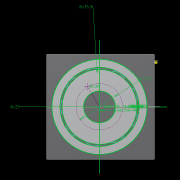
# Autodesk Inventor part: OuterBearingTest_TBS
Saved by Autodesk Inventor 2022.2 (Build 262287010, 287A)
## iProperties
Created: 2022-05-21
Part Number: OuterBearingTest_TBS
Material: Generic
Document SubType Name: Modeling
Designer: Árni Þór Þorgeirsson
Density: 1 g/cm^3
Appearance: Default
Author: Árni Þór Þorgeirsson
Autodesk Inventor part; units mm, degrees
ref_plane "YZ Plane" through (0, 0, 0) normal (1, 0, 0) x (0, 1, 0)
ref_plane "XZ Plane" through (0, 0, 0) normal (0, 1, 0) x (-1, 0, 0)
sketch "Sketch7" plane through (0, 0, 0) normal (0, 1, 0) x (-1, 0, 0)
  line L0 (0, 0) -> (0, 63.4182)
  line L1 (0, 0) -> (-60.766, 0) construction
  line L2 (0, 63.4182) -> (-60.766, 0) construction
  line L3 (0, 63.4182) -> (-66.3755, 0) construction
  line L4 (0, 63.4182) -> (-60.5189, -5.5956) construction
  line L5 (0, 0) -> (0, -63.4182)
  line L6 (0, -63.4182) -> (-60.766, 0) construction
  line L7 (0, -63.4182) -> (-66.3755, 0) construction
  line L8 (0, -63.4182) -> (-60.5189, 5.5956) construction
  line L9 (-60.5189, 5.5956) -> (-66.3755, 0) construction
  line L10 (-55.6121, 0) -> (-64.3632, -8.3612) construction
  line L11 (-55.6121, 0) -> (-39.6464, -15.2543) construction
  line L12 (0, -88.9988) -> (0, 125.9803) projected
  line L13 (-53.5, -5.9919) -> (-53.5, 6.008)
  line L14 (83.2786, 0) -> (-105.9214, 0) projected
  line L15 (-63.5667, 2.6836) -> (-57.9653, -2.6836) construction
  line L16 (-57.9653, 2.6836) -> (-63.5667, -2.6836) construction
  line L17 (-26.151, -15.9303) -> (-40.3783, -15.9303) construction
  line L18 (-40.3783, -15.9303) -> (-40.3783, -12.7539) construction
  line L19 (-40.3783, -12.7539) -> (-26.151, -12.7539) construction
  line L20 (-26.151, -12.7539) -> (-26.151, -15.9303) construction
  point P0 (-53.5, 0)
  dimension "Roller_Side_difference" = -0.164
  dimension "d90" = 63.4182
  dimension "d201" = 53.5
  dimension "d343" = 92.447
  dimension "d344" = 92.611
  dimension "d367" = 8.1
  constraints: 28 end point, 9 point on line, 3 midpoint, 3 vertical, 2 horizontal, 2 parallel, 2 perpendicular, 1 collinear, 1 symmetric about line, 2 other
  measures "d90" distance of L0.start L0.end
  measures "d201" distance between parallel lines of L5 L13
  measures "d343" angle of L10 L8
  measures "d344" angle of L7 L10
  measures "d367" distance of L3.end L8.end
sketch "Sketch1" plane through (0, 0, 0) normal (0, 0, 1) x (1, 0, 0)
  circle A0 centre (0, 0) radius 60.766 construction
  line L0 (0, 0) -> (60.766, 0)
  line L1 (0, 0) -> (60.766, 4.025)
  line L2 (60.766, 0) -> (60.766, 4.025)
  circle A1 centre (0, 0) radius 53.5
  point P0 (56.8, 0)
  dimension "d56" = 60.766
  dimension "d57" = 4.025
  dimension "d400" = 53.5
  dimension "d531" = 5.5
  dimension "d532" = 5.5
  dimension "d533" = 5.5
  dimension "d537" = 24.5
  dimension "d538" = 3
  dimension "d543" = 5
  dimension "d549" = 3
  dimension "d550" = 3
  dimension "d567" = 5
  dimension "d568" = 5
  constraints: 1 other
sketch "Roller1" plane through (0, 0, 0) normal (0, 1, 0) x (-1, 0, 0)
  line L0 (0, 63.4182) -> (-60.5189, -5.5956) construction
  line L1 (0, 63.4182) -> (-66.3755, 0) construction
  line L2 (-55.6121, 0) -> (-39.6464, -15.2543) construction
  line L3 (0, -63.4182) -> (-66.3755, 0) construction
  line L4 (-55.5642, 0.0925) -> (-60.471, -5.5031)
  line L5 (-60.471, -5.5031) -> (-66.285, 0.0519)
  line L6 (-66.285, 0.0519) -> (-60.9033, 5.1938)
  line L7 (-60.9033, 5.1938) -> (-55.5642, 0.0925)
  line L8 (-52.4316, -2.9004) -> (-57.5682, -8.2765)
  line L9 (-53.1547, -2.2096) -> (-58.2912, -7.5857)
  point P0 (0, 0)
  point P1 (-63.378, -2.7256)
  dimension "d345" = 0.025
  dimension "d346" = 0.025
  dimension "d347" = 0.1
  dimension "d348" = 0.1
  dimension "d349" = 272.61
  dimension "d350" = 272.447
  dimension "d357" = 1
  dimension "d369" = 4.0148
  constraints: 12 end point, 5 parallel, 4 point on line, 1 midpoint, 1 perpendicular
  measures "d345" distance between parallel lines of L0 L4
  measures "d346" distance between parallel lines of L1 L6
  measures "d347" distance between parallel lines of L3 L5
  measures "d348" distance between parallel lines of L2 L7
  measures "d357" distance between parallel lines of L8 L9
  measures "d369" distance from line of L4.end L8
sketch "Roller2" plane through (0, 0, 0) normal (0, 1, 0) x (-1, 0, 0)
  line L0 (0, -63.4182) -> (-60.5189, 5.5956) construction
  line L1 (-55.6121, 0) -> (-64.3632, -8.3612) construction
  line L2 (0, -63.4182) -> (-66.3755, 0) construction
  line L3 (0, 63.4182) -> (-66.3755, 0) construction
  line L4 (-60.471, 5.5031) -> (-55.6961, 0.058)
  line L5 (-55.6961, 0.058) -> (-61.048, -5.0555)
  line L6 (-61.048, -5.0555) -> (-66.285, -0.0519)
  line L7 (-66.285, -0.0519) -> (-60.471, 5.5031)
  line L8 (-63.378, 2.7256) -> (-58.3796, -2.5059)
  line L9 (-62.655, 3.4164) -> (-57.6565, -1.8151)
  point P0 (0, 0)
  dimension "d351" = 0.025
  dimension "d352" = 0.025
  dimension "d354" = 0.1
  dimension "d355" = 92.447
  dimension "d356" = 92.611
  dimension "d370" = 0.1
  dimension "d371" = 1
  constraints: 12 end point, 5 parallel, 3 point on line, 1 midpoint, 1 perpendicular
  measures "d351" distance between parallel lines of L0 L4
  measures "d352" distance between parallel lines of L2 L6
  measures "d354" distance between parallel lines of L1 L5
  measures "d355" angle of L5 L4
  measures "d356" angle of L6 L5
  measures "d370" distance from line of L3 L8.start
  measures "d371" distance between parallel lines of L9 L8
sketch "Sketch22" plane through (0, 0, 0) normal (0, 1, 0) x (-1, 0, 0)
  line L0 (-31.756, 8.0215) -> (-17.5287, 8.0215) construction
  line L1 (-17.5287, 8.0215) -> (-17.5287, 4.8451) construction
  line L2 (-17.5287, 4.8451) -> (-31.756, 4.8451) construction
  line L3 (-31.756, 4.8451) -> (-31.756, 8.0215) construction
  point P0 (0, 0)
  dimension "Roller_Side_difference" = -0.164
  constraints: 2 other
sketch "Sketch2" plane through (0, 0, 0) normal (0, 1, 0) x (-1, 0, 0)
  line L0 (0, 0) -> (0, 60.766) construction
  line L1 (0, 0) -> (-60.766, 0) projected
  line L2 (0, 0) -> (0, -60.766)
  line L3 (0, -60.766) -> (-60.766, 0) construction
  line L4 (0, 60.766) -> (-60.766, 0) construction
  line L5 (-78.8928, 100.3938) -> (0, 60.766) construction
  line L6 (-36.7785, 14.3639) -> (0, 60.766) construction
  line L7 (-36.7785, 14.3639) -> (0, -60.766) construction
  line L8 (-39.0257, 11.5288) -> (0, -60.766) construction
  point P0 (-41.1854, 19.5806)
  constraints: 16 end point, 3 point on line, 1 perpendicular, 1 symmetric about line, 1 vertical
sketch "Sketch23" plane through (0, 0, 0) normal (0, 1, 0) x (-1, 0, 0)
  line L0 (0, -63.4182) -> (-60.5189, 5.5956) construction
  line L1 (0, -63.4182) -> (-66.3755, 0) construction
  line L2 (0, 63.4182) -> (-60.5189, -5.5956) construction
  line L3 (-60.5189, 5.5956) -> (-66.3755, 0) construction
  line L4 (0, 63.4182) -> (-66.3755, 0) construction
  line L5 (-60.5189, 5.5956) -> (-60.5189, -5.5956) construction
  line L6 (83.2786, 0) -> (-105.9214, 0) projected
  line L7 (-59.0705, 4.0956) -> (-55.5369, 0.0659)
  line L8 (-55.5369, -0.0659) -> (-59.0705, -4.0956)
  line L9 (-62.2336, 4.0956) -> (-66.4445, 0.0723)
  line L10 (-66.4445, -0.0723) -> (-62.2336, -4.0956)
  arc A0 (-66.4445, 0.0723) -> (-66.4445, -0.0723) centre (-66.3755, 0) ccw
  arc A1 (-55.5369, -0.0659) -> (-55.5369, 0.0659) centre (-55.6121, 0) ccw
  line L11 (-59.0705, 4.0956) -> (-59.0705, 5.5956)
  line L12 (-59.0705, 5.5956) -> (-25, 5.5956)
  line L13 (-25, 5.5956) -> (-25, -5.5956)
  line L14 (-25, -5.5956) -> (-59.0705, -5.5956)
  line L15 (-59.0705, -5.5956) -> (-59.0705, -4.0956)
  line L16 (-62.2336, 4.0956) -> (-62.2336, 5.5956)
  line L17 (-62.2336, 5.5956) -> (-75, 5.5956)
  line L18 (-75, 5.5956) -> (-75, -5.5956)
  line L19 (-62.2336, -4.0956) -> (-62.2336, -5.5956)
  line L20 (-62.2336, -5.5956) -> (-75, -5.5956)
  line L21 (-60.5189, 5.5956) -> (-60.5189, 5.5956)
  line L22 (-60.5189, -5.5956) -> (-60.5189, -5.5956)
  line L23 (0, -88.9988) -> (0, 125.9803) projected
  line L24 (-66.5202, 0) -> (-75, 0)
  point P0 (0, 0)
  point P1 (-55.4791, 0)
  point P2 (-66.4755, 0)
  point P3 (-75, 0)
  dimension "d378" = 90
  dimension "d379" = 0.1
  dimension "d380" = 0.1
  dimension "d381" = 0.1
  dimension "d382" = 0.1
  dimension "d383" = 0.1
  dimension "d384" = 11.1912
  dimension "d385" = 0
  dimension "d386" = 0
  dimension "d391" = 25
  dimension "d392" = 75
  dimension "d393" = 1.5
  dimension "d394" = 1.5
  dimension "d395" = 1.5
  dimension "d396" = 1.5
  constraints: 36 end point, 10 point on line, 9 vertical, 4 horizontal, 4 parallel, 4 point on circle, 4 tangent, 2 centre point, 1 equal radius, 1 midpoint
  measures "d378" angle of L6 L5
  measures "d379" radius of A0
  measures "d380" distance between parallel lines of L9 L4
  measures "d381" distance between parallel lines of L10 L1
  measures "d382" distance between parallel lines of L0 L7
  measures "d383" distance between parallel lines of L2 L8
  measures "d384" distance of L0.end L2.end
  measures "d385" distance of L2.end L22.end
  measures "d386" distance of L0.end L21.end
  measures "d391" distance between parallel lines of L23 L13
  measures "d392" distance between parallel lines of L18 L23
  measures "d393" distance of L9.start L16.end
  measures "d394" distance of L7.start L11.end
  measures "d395" distance of L14.end L8.end
  measures "d396" distance of L10.end L19.end
revolve "RevRoller1" [suppressed]
fillet "Fillet1" [suppressed]
sketch "Sketch40" plane through (0, 0, -5.5956) normal (0, 0, -1) x (-1, 0, 0)
  circle A0 centre (75, 0) radius 2.5 projected
  circle A1 centre (0, 0) radius 53.5 projected
  point P0 (53.4416, 2.4993)
  point P1 (53.4416, -2.4993)
sketch "Sketch43" plane through (0, 0, 20) normal (0, 0, 1) x (1, 0, 0)
  circle A0 centre (0, 0) radius 14.9199 projected
  circle A1 centre (0, 0) radius 70.1809
  circle A2 centre (0, 0) radius 22.9199
  circle A3 centre (0, 0) radius 21.1699
  circle A4 centre (-21.1699, 0) radius 1.5
  circle A5 centre (21.4375, -37.1308) radius 1.5 projected
  circle A6 centre (15.3125, 26.522) radius 1.5 projected
  circle A7 centre (0, 0) radius 1 projected
  circle A8 centre (15.3125, 26.522) radius 1.5 projected
  line L0 (0, 0) -> (35.0904, 60.7784)
  line L1 (0, 0) -> (35.0904, -60.7784)
  circle A9 centre (-30.625, 0) radius 2.5 projected
  line L2 (-21.1699, -8.7839) -> (-21.1699, 8.7839)
  circle A10 centre (-30.625, 0) radius 4.5
  arc A11 (-30.625, 4.5) -> (-21.1699, 8.7839) centre (-30.3626, 16.4971) ccw
  arc A12 (-21.1699, -8.7839) -> (-30.625, -4.5) centre (-30.3626, -16.4971) ccw
  circle A13 centre (21.1699, 0) radius 1.5
  line L3 (21.1699, 8.7839) -> (21.1699, -8.7839)
  circle A14 centre (30.625, 0) radius 4.5
  arc A15 (30.625, -4.5) -> (21.1699, -8.7839) centre (30.3626, -16.4971) ccw
  arc A16 (21.1699, 8.7839) -> (30.625, 4.5) centre (30.3626, 16.4971) ccw
  point P0 (-30.4819, -4.4977)
  point P1 (-30.4819, 4.4977)
  point P2 (11.46, 19.8492)
  point P3 (14.5625, 25.223)
  point P4 (16.0625, 27.8211)
  point P5 (22.1875, -38.4299)
  point P6 (20.6875, -35.8318)
  point P7 (11.46, -19.8492)
  point P8 (30.4819, -4.4977)
  point P9 (30.4819, 4.4977)
  dimension "d585" = 8
  dimension "d587" = 1.75
  dimension "d589" = 3
  dimension "d592" = 2
  dimension "d593" = 12
  dimension "d594" = 12
  dimension "d597" = 3
  dimension "d598" = 12
  dimension "d599" = 12
  constraints: 16 point on circle, 10 centre point, 8 end point, 2 midpoint, 1 horizontal alignment, 1 vertical, 2 other
  measures "d585" radial gap between concentric circles of A0 A2
  measures "d589" diameter of A4
  measures "d592" radial gap between concentric circles of A9 A10
  measures "d593" radius of A11
  measures "d594" radius of A12
  measures "d597" diameter of A13
  measures "d598" radius of A15
  measures "d599" radius of A16
pattern_circular "Circular Pattern13" [suppressed]
feature "Move Body7" [suppressed]
revolve "Revolution13" [suppressed]
fillet "Fillet3" [suppressed]
pattern_circular "Circular Pattern14" [suppressed]
feature "Move Body6" [suppressed]
revolve "Revolution14" add sketch "Sketch23" angle 360 about axis through (0, 0, -10) along (0, 0, 1) contours A1 L7 L11 L12 L13 L6 | L6 L13 L14 L15 L8 A1
revolve "OuterRim_Top2" add sketch "Sketch23" angle 360 about axis through (0, 0, -10) along (0, 0, 1) contours L6 A0 L10 L19 L20 L18
revolve "OuterRim_Bottom2" add sketch "Sketch23" angle 360 about axis through (0, 0, -10) along (0, 0, 1) contours L6 L18 L17 L16 L9 A0
sketch "Sketch30" plane through (0, 0, 5.5956) normal (0, 0, 1) x (1, 0, 0)
  circle A0 centre (0, 0) radius 25 projected
  line L0 (0, 0) -> (2.5, 0)
  circle A1 centre (2.5, 0) radius 4
  dimension "d495" = 2.5
  dimension "d496" = 8
  constraints: 2 end point, 1 centre point, 1 coincident, 1 horizontal
  measures "d495" distance of L0.start L0.end
  measures "d496" diameter of A1
ref_plane "Work Plane7" through (0, 0, 100) normal (0, 0, 1) x (1, 0, 0)
sketch "Sketch44" plane through (0, 0, 100) normal (0, 0, 1) x (1, 0, 0)
  circle A0 centre (0, 0) radius 75 projected
  circle A1 centre (0, 0) radius 62.2336 projected
  circle A2 centre (0, 0) radius 59.0705 projected
  circle A3 centre (0, 0) radius 25 projected
  line L0 (0, 0) -> (-18.375, 31.8264) construction
  line L1 (0, -105) -> (0, 105) projected
  circle A4 centre (0, 0) radius 36.75 construction
  dimension "d604" = 73.5
  dimension "d603" = 30
  constraints: 2 coincident, 2 end point, 3 other
  measures "d603" angle of L1 L0
equation "\"Roller_Side_difference\" = -0.163578deg"
equation "\"Cycloid_Top_Plate_Fasner_Inner\" = 61.25"
equation "\"Cycloid_Top_Plate_Fasner_Outer\" = 85.75"
equation "\"Roller_Hole_Radius\" = 1"
equation "\"Distance_To_Bearing\" = 87.83151"
equation "\"Bearing_Roller_Gap_Reduction\" = 0.2"
equation "\"d514\" = 0.2"
equation "\"Side_Bearing_Outer_Diameter\" = 75"
equation "\"Side_Bearing_Inner_Diameter\" = 25"
body "Solid1"
body "Solid5"
